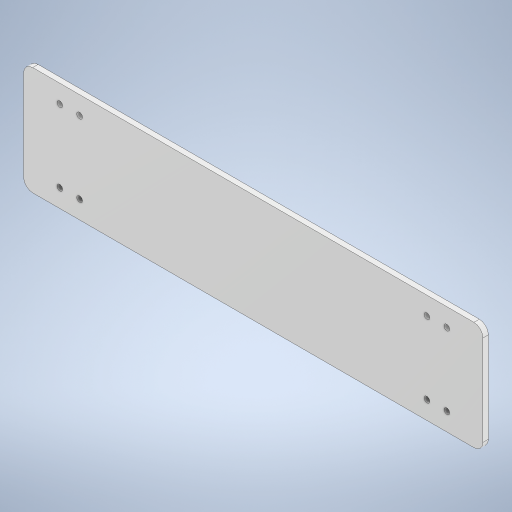
# Autodesk Inventor part: BP_BOX-Back-60
Saved by Autodesk Inventor 2024.3 (Build 283343000, 343)
## iProperties
Created: 2025-04-19
Part Number: BP_BOX-Back-60
Material: アセタール樹脂、白
Document SubType Name: Modeling
Designer: ngt-a
Density: 1.425 g/cm^3
Appearance: 滑らか - 白
Mass: 67.1611 g
Surface Area: 355.524 cm^2
Volume: 51.268 cm^3
Author: ngt-a
Autodesk Inventor part; units mm, degrees
ref_plane "YZ Plane" through (0, 0, 0) normal (1, 0, 0) x (0, 1, 0)
ref_plane "XZ Plane" through (0, 0, 0) normal (0, 1, 0) x (-1, 0, 0)
ref_plane "XY Plane" through (0, 0, 0) normal (0, 0, 1) x (1, 0, 0)
sketch "スケッチ1" plane through (0, 0, 0) normal (0, 1, 0) x (-1, 0, 0)
  line L0 (130, 1.5) -> (-130, 1.5)
  line L1 (-130, 1.5) -> (-130, -1.5)
  line L2 (-130, -1.5) -> (130, -1.5)
  line L3 (130, -1.5) -> (130, 1.5)
  line L4 (130, 1.5) -> (-130, -1.5) construction
  line L5 (-130, 1.5) -> (130, -1.5) construction
  point P0 (0, 0)
  dimension "d0" = 260
  dimension "d1" = 3
  constraints: 12 end point, 2 midpoint, 2 parallel, 1 horizontal, 1 perpendicular
  measures "d0" distance of L1.end L2.end
  measures "d1" distance of L2.end L0.start
extrude "押し出し1" add sketch "スケッチ1" along normal blind 60
sketch "スケッチ5" plane through (130, 0, -1.5) normal (0, 0, -1) x (-1, 0, 0)
  line L0 (0, 0) -> (260, 0) projected
  line L1 (0, 60) -> (3, 60)
  line L2 (3, 60) -> (3, 0)
  line L3 (3, 0) -> (0, 0)
  line L4 (0, 0) -> (0, 60)
  line L5 (0, 45) -> (3, 45)
  line L6 (3, 45) -> (3, 15)
  line L7 (3, 15) -> (0, 15)
  line L8 (0, 15) -> (0, 45)
  line L9 (0, 60) -> (260, 60) projected
  line L10 (130, 60) -> (130, 0)
  line L11 (260, 0) -> (0, 0)
  line L12 (260, 60) -> (257, 60)
  line L13 (257, 60) -> (257, 0)
  line L14 (260, 0) -> (260, 60)
  line L15 (260, 45) -> (257, 45)
  line L16 (257, 15) -> (260, 15)
  point P0 (1.5, 45)
  point P1 (1.5, 60)
  point P2 (1.5, 15)
  point P3 (1.5, 0)
  point P4 (258.5, 15)
  point P5 (257, 0)
  point P6 (257, 60)
  point P7 (0, 15)
  point P8 (3, 45)
  dimension "d22" = 3
  dimension "d23" = 15
  dimension "d24" = 15
  constraints: 30 end point, 10 symmetric about line, 6 point on line, 5 midpoint, 4 parallel, 3 perpendicular, 2 horizontal
  measures "d22" distance between parallel lines of L2 L4
  measures "d23" distance of point (1.5, 45) point (1.5, 60)
  measures "d24" distance of point (1.5, 15) point (1.5, 0)
extrude "押し出し4" cut sketch "スケッチ5" against normal through all contours L4 L7 L2 L0 | L4 L5 L2 L7 | L4 L1 L2 L5 | L13 L16 L14 L0 | L13 L15 L14 L16 | L9 L14 L15 L13
sketch "スケッチ8" plane through (-127, 0, 1.5) normal (0, 0, 1) x (1, 0, 0)
  circle A0 centre (20, 50) radius 1.6
  circle A1 centre (20, 10) radius 1.6
  line L0 (0, 60) -> (0, 0) projected
  line L1 (0, 60) -> (254, 60) projected
  line L2 (0, 0) -> (254, 0) projected
  line L3 (127, 60) -> (127, 0)
  circle A2 centre (234, 50) radius 1.6
  circle A3 centre (234, 10) radius 1.6
  dimension "d31" = 20
  dimension "d32" = 10
  dimension "d33" = 20
  dimension "d34" = 10
  dimension "d35" = 3.2
  dimension "d36" = 3.2
  constraints: 4 centre point, 2 end point, 2 symmetric about line, 1 midpoint, 1 vertical, 2 other
  measures "d31" distance from line of A0.centre L0
  measures "d32" distance from line of A0.centre L1
  measures "d33" distance from line of A1.centre L0
  measures "d34" distance from line of L2 A1.centre
  measures "d35" diameter of A0
  measures "d36" diameter of A1
extrude "押し出し7" cut sketch "スケッチ8" against normal through all contours A0 | A1 | A2 | A3
fillet "フィレット1" radius 5 4 edges at (-127, 60, 0) (-127, 0, 0) (127, 60, 0) (127, 0, 0)
sketch "スケッチ13" plane through (-122, 0, 1.5) normal (0, 0, 1) x (1, 0, 0)
  line L0 (244, 60) -> (0, 60) projected
  line L1 (122, 60) -> (122, 0)
  circle A0 centre (15, 50) radius 1.6 projected
  circle A1 centre (15, 10) radius 1.6 projected
  point P0 (26, 50)
  point P1 (26, 10)
  point P2 (218, 50)
  point P3 (218, 10)
  dimension "d60" = 11
  dimension "d61" = 11
  dimension "d62" = 40
  dimension "d63" = 10
  constraints: 2 end point, 2 symmetric about line, 1 midpoint, 1 vertical
  measures "d60" distance of A0.centre point (26, 50)
  measures "d61" distance of A1.centre point (26, 10)
  measures "d62" distance of point (26, 10) point (26, 50)
  measures "d63" distance from line of L0 point (26, 50)
hole "穴1" at (-96, 50, 1.5) at (-96, 10, 1.5) at (96, 50, 1.5) at (96, 10, 1.5) direction (0, 0, -1) diameter 3.2 end through all
equation "\"d36\" = d35"
equation "\"d61\" = d60"
